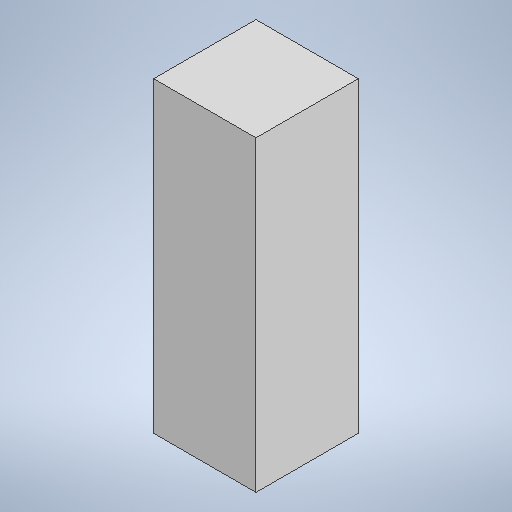
# Autodesk Inventor part: Flocculant barrel
Saved by Autodesk Inventor 2025 (Build 290162010, 162A)
## iProperties
Created: 2025-03-29
Part Number: Flocculant barrel
Material: Generic
Document SubType Name: Modeling
Designer: pokla
Density: 1 g/cm^3
Appearance: Default
Author: pokla
Autodesk Inventor part; units mm, degrees
ref_plane "YZ Plane" through (0, 0, 0) normal (1, 0, 0) x (0, 1, 0)
ref_plane "XZ Plane" through (0, 0, 0) normal (0, 1, 0) x (-1, 0, 0)
ref_plane "XY Plane" through (0, 0, 0) normal (0, 0, 1) x (1, 0, 0)
sketch "Sketch1" plane through (0, 0, 0) normal (0, 0, 1) x (1, 0, 0)
  line L0 (-200, -200) -> (200, -200)
  line L1 (200, -200) -> (200, 200)
  line L2 (200, 200) -> (-200, 200)
  line L3 (-200, 200) -> (-200, -200)
  line L4 (200, -200) -> (-200, 200) construction
  point P0 (0, 0)
  point P1 (0, 0)
  dimension "d0" = 400
  dimension "d1" = 400
  constraints: 10 end point, 2 parallel, 1 coincident, 1 horizontal, 1 midpoint, 1 perpendicular
  measures "d0" distance of L2.end L0.start
  measures "d1" distance between parallel lines of L1 L3
extrude "Extrusion1" add sketch "Sketch1" along normal blind 1200
equation "\"d0\" = Длина"
equation "\"d1\" = Ширина"
equation "\"d2\" = Высота"
equation "\"Длина\" = 400"
equation "\"Ширина\" = 400"
equation "\"Высота\" = 1200"
body "Solid1"
